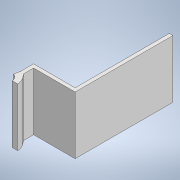
# Autodesk Inventor part: prototype_12_cover
Saved by Autodesk Inventor 2022 (Build 260153000, 153)
## iProperties
Created: 2022-06-23
Part Number: prototype_12_cover
Material: Generic
Document SubType Name: Modeling
Designer: tecware
Density: 1 g/cm^3
Appearance: Default
Author: tecware
Autodesk Inventor part; units mm, degrees
ref_plane "YZ Plane" through (0, 0, 0) normal (1, 0, 0) x (0, 1, 0)
ref_plane "XZ Plane" through (0, 0, 0) normal (0, 1, 0) x (-1, 0, 0)
ref_plane "XY Plane" through (0, 0, 0) normal (0, 0, 1) x (1, 0, 0)
sketch "Sketch1" plane through (0, 0, 0) normal (0, 1, 0) x (-1, 0, 0)
  line L0 (-0.0003, 59.6701) -> (0.6603, 62.5452) projected
  line L1 (-2.25, 66.2) -> (-5.2, 66.2) projected
  line L2 (0, 19.4) -> (-7, 19.4)
  line L3 (-7, 19.4) -> (-7, 35.6)
  line L4 (-7, 35.6) -> (0, 35.6)
  arc A0 (0.6603, 62.5452) -> (-2.25, 66.2) centre (1.5, 66.2) ccw projected
  arc A1 (3, 59.6701) -> (-5.2, 66.2) centre (1.5, 66.2) ccw projected
  arc A2 (0.6603, 62.5452) -> (-2.25, 66.2) centre (1.5, 66.2) ccw projected
  line L5 (0, 35.6) -> (0, 59.6701) projected
  line L6 (1.5, 66.2) -> (-2.25, 66.2)
  line L7 (1.5, 66.2) -> (0.6603, 62.5452)
  line L8 (1.5, 66.2) -> (-5.2118, 66.0064)
  arc A3 (-2.2484, 66.0919) -> (0.5552, 62.571) centre (1.5, 66.2) ccw
  line L9 (-0.2, 52.3701) -> (-23, 52.3701)
  line L10 (-25, 54.1701) -> (-2.2, 54.1701)
  line L11 (-23, 2.2) -> (-23, 52.3701)
  line L12 (0, 0) -> (0, 19.4) projected
  line L13 (-24.1293, 0) -> (0, 0) projected
  line L14 (-25, 0) -> (-24.1293, 0) projected
  line L15 (-25, 0.2) -> (-0.2, 0.2)
  line L16 (-0.2, 0.2) -> (-0.2, 2.2)
  line L17 (-0.2, 2.2) -> (-23, 2.2)
  line L18 (-25, 0.2) -> (-25, 54.1701)
  line L19 (-23, 2.2) -> (-23, 0.2)
  circle A4 centre (1.5, 66.2) radius 6.7
  line L20 (-0.2, 52.3701) -> (-0.2, 59.7193)
  line L21 (0.5552, 62.571) -> (-0.2, 59.7193)
  line L22 (-2.2, 54.1701) -> (-2.2, 60.6143)
  point P0 (-5.1972, 66.0068)
  dimension "d14" = 1.652
  dimension "d18" = 22.8
  dimension "d21" = 24.8
  dimension "d22" = 0.2
  dimension "d23" = 2
  constraints: 35 end point, 5 point on circle, 4 point on line, 2 centre point, 1 coincident, 1 parallel, 1 perpendicular, 2 other
  measures "d14" angle of L6 L8
  measures "d18" distance of L10.start L10.end
  measures "d21" distance of L15.start L15.end
  measures "d22" distance between parallel lines of L13 L15
  measures "d23" distance of L15.end L16.end
extrude "Extrusion1" add sketch "Sketch1" along normal mid plane 32 contours L20 L9 L11 L19 L15 L18 L10 L22 A4 | A4 L8 A3 L21
sketch "Sketch2" plane through (0, -16, 0) normal (0, -1, 0) x (1, 0, 0)
  spline S0 degree 3 poles (24.1293, 0) (23.5574, -0.0479) (22.9856, -0.0965) (22.4138, -0.1456) (19.2606, -0.4164) (16.108, -0.6985) (8.6399, -1.2015) (4.3202, -1.3606) (0, -1.3606) (-4.3202, -1.3606) (-8.6399, -1.2015) (-16.108, -0.6985) (-19.2606, -0.4164) (-22.4138, -0.1456) (-23.2758, -0.0716) (-24.1378, 0.0014) (-25, 0.0722) knots -0.172158 -0.172158 -0.172158 -0.172158 0 0 0 0.949465 0.949465 2.245518 2.245518 2.245518 3.54157 3.54157 4.491036 4.491036 4.491036 4.750564 4.750564 4.750564 4.750564 projected
  line L0 (24.1293, 0) -> (0, 0) projected
  line L1 (0, 0) -> (0, 19.4) projected
  line L2 (0, 19.4) -> (7, 19.4) projected
  line L3 (7, 35.6) -> (7, 19.4) projected
  line L4 (0, 35.6) -> (7, 35.6) projected
  line L5 (0, 35.6) -> (0, 59.6701) projected
  arc A0 (0, 59.6701) -> (0.0003, 59.6701) centre (-1.5, 66.2) ccw projected
  line L6 (0.0003, 59.6701) -> (-0.6603, 62.5452) projected
  arc A1 (2.25, 66.2) -> (-0.6603, 62.5452) centre (-1.5, 66.2) ccw projected
  line L7 (2.25, 66.2) -> (5.2, 66.2) projected
  arc A2 (5.2, 66.2) -> (-3, 59.6701) centre (-1.5, 66.2) ccw projected
  line L8 (-3, 59.6701) -> (-3, 4.75) projected
  line L9 (-25, 4.75) -> (-3, 4.75) projected
  line L10 (-25, 0.0722) -> (-25, 4.75) projected
  line L11 (0, 21.4) -> (6, 21.4) projected
  line L12 (0, 21.4) -> (0, 33.6) projected
  line L13 (0, 33.6) -> (6, 33.6) projected
  line L14 (6, 33.6) -> (6, 21.4) projected
  line L15 (0, 35.8) -> (7.2, 35.8)
  line L16 (7.2, 35.8) -> (7.2, 19.2)
  line L17 (7.2, 19.2) -> (0, 19.2)
  line L18 (0, 19.2) -> (0, 35.8)
  line L19 (0.2, 52.3701) -> (23, 52.3701) projected
  line L20 (0.2, 52.3701) -> (0.2, 35.8)
  line L21 (0.2, 19.2) -> (0.2, 0.2)
  line L22 (23, 0.2) -> (25, 0.2) projected
  line L23 (23, 52.3701) -> (23, 0.2) projected
  line L24 (0.2, 0.2) -> (23, 0.2)
  dimension "d24" = 7.2
  dimension "d25" = 16.6
  dimension "d26" = 0.2
  dimension "d27" = 0.2
  constraints: 14 end point, 3 point on line, 2 parallel, 1 collinear
  measures "d24" distance of L16.end L17.end
  measures "d25" distance of L15.end L16.end
  measures "d26" distance between parallel lines of L4 L15
  measures "d27" distance between parallel lines of L1 L21
extrude "Extrusion2" add sketch "Sketch2" against normal blind 2 contours L17 L16 L15 L20 L19 L23 L24 L21
equation "\"d14\" = d17"
equation "\"d17\" = 1.652443deg"
body "Solid1"
